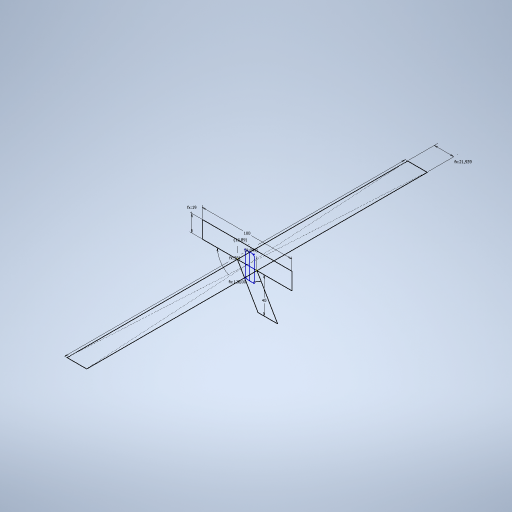
# Autodesk Inventor part: Clamex Joint1100
Saved by Autodesk Inventor 2024 (Build 280153000, 153)
## iProperties
RuleStatus: InUse
Created: 2023-01-09
Part Number: Clamex Joint1100
Material: Generic
Document SubType Name: Modeling
Designer: sauliusd
Density: 1 g/cm^3
Appearance: Default
AfterAnyUserParamChange0: ComponentsArrayParams
Author: sauliusd
Autodesk Inventor part; units mm, degrees
ref_plane "YZ Plane" through (0, 0, 0) normal (1, 0, 0) x (0, 1, 0)
ref_plane "XZ Plane" through (0, 0, 0) normal (0, 1, 0) x (-1, 0, 0)
ref_plane "XY Plane" through (0, 0, 0) normal (0, 0, 1) x (1, 0, 0)
sketch "Sketch1" plane through (0, 0, 0) normal (0, 0, 1) x (1, 0, 0)
  line L0 (-190.5, -10.9695) -> (190.5, -10.9695)
  line L1 (190.5, -10.9695) -> (190.5, 10.9695)
  line L2 (190.5, 10.9695) -> (-190.5, 10.9695)
  line L3 (-190.5, 10.9695) -> (-190.5, -10.9695)
  line L4 (-190.5, -10.9695) -> (190.5, 10.9695) construction
  line L5 (190.5, -10.9695) -> (-190.5, 10.9695) construction
  point P0 (0, 0)
  dimension "d0" = 381
  dimension "d1" = 21.939
  constraints: 12 end point, 2 midpoint, 2 parallel, 1 horizontal, 1 perpendicular
  measures "d0" distance of L2.end L1.end
  measures "d1" distance of L0.end L1.end
sketch "Lamello" plane through (0, 0, 0) normal (0, 0, 1) x (1, 0, 0)
  line L0 (48.383, 141.1858) -> (42.783, 141.1858)
  line L1 (40.583, 139.6858) -> (40.583, 114.6858)
  line L2 (42.783, 113.1858) -> (48.383, 113.1858)
  line L3 (50.583, 114.6858) -> (50.583, 139.6858)
  line L4 (50.583, 139.6858) -> (48.383, 141.1858)
  line L5 (40.583, 139.6858) -> (42.783, 141.1858)
  line L6 (40.583, 114.6858) -> (42.783, 113.1858)
  line L7 (50.583, 114.6858) -> (48.383, 113.1858)
  line L8 (50.583, 127.1858) -> (40.583, 127.1858)
  line L9 (45.583, 141.1858) -> (45.583, 113.1858)
  point P0 (45.583, 127.1858)
  point P1 (50.583, 141.1858)
  point P2 (40.583, 113.1858)
  point P3 (40.583, 141.1858)
  point P4 (50.583, 113.1858)
  dimension "d54" = 10
  dimension "d55" = 28
  dimension "d56" = 1.5
  dimension "d57" = 2.2
  dimension "d58" = 1.5
  dimension "d59" = 2.2
  dimension "d60" = 1.5
  dimension "d61" = 2.2
  dimension "d62" = 1.5
  dimension "d63" = 2.2
  measures "d54" distance of point (50.583, 113.186) point (40.583, 113.186)
  measures "d55" distance of point (40.583, 113.186) point (40.583, 141.186)
  measures "d56" distance of L3.end point (50.583, 141.186)
  measures "d57" distance of L0.start point (50.583, 141.186)
  measures "d58" distance of L1.start point (40.583, 141.186)
  measures "d59" distance of L0.end point (40.583, 141.186)
  measures "d60" distance of L1.end point (40.583, 113.186)
  measures "d61" distance of L2.start point (40.583, 113.186)
  measures "d62" distance of L3.start point (50.583, 113.186)
  measures "d63" distance of L2.end point (50.583, 113.186)
sketch "Sketch2" plane through (0, 0, 0) normal (0, 0, 1) x (1, 0, 0)
  circle A0 centre (130.5, 3.7778) radius 0.5
  line L0 (190.5, 10.9695) -> (-190.5, 10.9695) projected
  line L1 (-190.5, -10.9695) -> (190.5, -10.9695) projected
  line L2 (0, -145.0303) -> (0, 106.9697) projected
  line L3 (190.5, -10.9695) -> (190.5, 10.9695) projected
  point P0 (0, 0)
  dimension "d4" = 1
  dimension "d50" = 7.1917
  dimension "d70" = 60
  constraints: 1 centre point
  measures "d4" diameter of A0
  measures "d50" distance from line of L0 A0.centre
  measures "d70" distance from line of L3 A0.centre
extrude "Extrusion1" add sketch "Sketch2" along normal blind 10 contours A0
pattern_linear "Clamex Array" count 2 spacing 261 along (-1, 0, 0) of "Extrusion1"
sketch "Edge-Side Connection" plane through (0, 0, 0) normal (1, 0, 0) x (0, 1, 0)
  line L0 (-50, 0) -> (50, 0)
  line L1 (50, 0) -> (50, 19)
  line L2 (50, 19) -> (-50, 19)
  line L3 (-50, 19) -> (-50, 0)
  line L4 (-10.9695, 0) -> (-34.0635, -40)
  line L5 (-34.0635, -40) -> (-12.1245, -40)
  line L6 (-12.1245, -40) -> (10.9695, 0)
  line L7 (-2.9208, -14) -> (-2.9208, 14) construction
  line L8 (10.9695, 0) -> (2.0792, 0)
  line L9 (-7.9208, -12.5) -> (-15.62, -8.0549)
  point P0 (0, 0)
  point P1 (10.9695, 0)
  point P2 (0, 0)
  dimension "d26" = 100
  dimension "d27" = 19
  dimension "d28" = 40
  dimension "OtherSideRefYCoordinate" = 8.0487
  dimension "ReferenceCoord" = 13.8903
  dimension "d49" = 120
  constraints: 20 end point, 3 horizontal, 3 parallel, 2 perpendicular, 2 point on line, 1 coincident, 1 equal length, 1 midpoint, 1 vertical, 2 other
  measures "d26" distance of L2.end L1.end
  measures "d27" distance of L1.end L0.end
  measures "d28" distance between parallel lines of L0 L5
  measures "OtherSideRefYCoordinate" distance from line of point (-10.969, 0) L7
  measures "ReferenceCoord" distance from line of point (10.97, 0) L7
  measures "d49" angle of L6 L0
sketch "Edge-Edge Connection" plane through (0, 0, 0) normal (1, 0, 0) x (0, 1, 0)
  line L0 (-109.0303, 19) -> (10.9697, 19)
  line L1 (10.9697, 19) -> (0, 0)
  line L2 (0, 0) -> (-109.0303, 0)
  line L3 (-109.0303, 0) -> (-109.0303, 19)
  line L4 (10.9697, 19) -> (70.9697, -84.923)
  line L5 (0, 0) -> (54.5152, -94.423)
  line L6 (54.5152, -94.423) -> (70.9697, -84.923)
  line L7 (1.0958, 1.8981) -> (0, 0)
  line L8 (-4.7295, 16.8083) -> (-4.7295, 19)
  point P0 (3.5958, 6.2282)
  dimension "d51" = 19
  dimension "d53" = 19
  dimension "EdgeEdgeReferenceCoord" = 7.1917
  dimension "d65" = 120
  dimension "d66" = 120
  dimension "d67" = 120
  dimension "EdgeEdgeOtherSideRefYCoordinate" = 14.7476
  constraints: 18 end point, 3 perpendicular, 2 parallel, 2 point on line, 1 coincident, 1 collinear, 1 equal length, 1 horizontal, 4 other
  measures "d51" distance between parallel lines of L2 L0
  measures "d53" distance between parallel lines of L4 L5
  measures "d65" angle of L2 L5
  measures "d66" distance of L0.start L0.end
  measures "d67" distance of L0.end L4.end
equation "\"d9\" = Step"
equation "\"d27\" = NestleBoardT"
equation "\"d0\" = ContactPatchWidth"
equation "\"d1\" = ContactPatchHeight"
equation "\"ContactPatchWidth\" = 381"
equation "\"ContactPatchHeight\" = 21.939"
equation "\"PlacingWidth\" = 261"
equation "\"MinDistBetween\" = 96"
equation "\"Step\" = 261"
equation "\"Y_Coord\" = 7.19169"
equation "\"NestleBoardT\" = 19"
equation "\"PillarBoardT\" = 19"
equation "\"AngleForYPositionCalc\" = 120deg"
equation "\"ConnectionAngle\" = 120deg"
